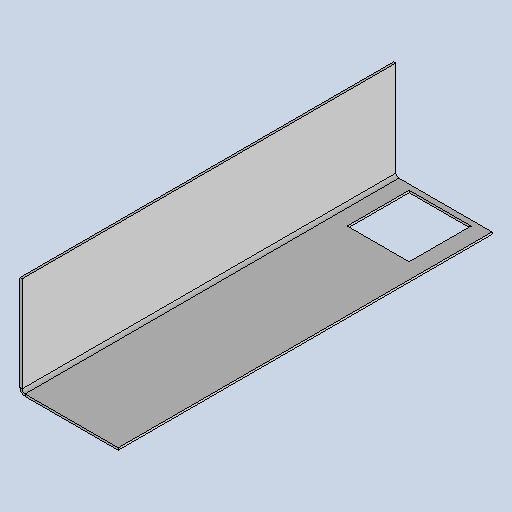
# Autodesk Inventor part: PNS 752 FDS 1200 FLANGE 2_1600
Saved by Autodesk Inventor 2025 (Build 290162010, 162A)
## iProperties
Created: 2025-06-24
Part Number: PNS 752 FDS 1200 FLANGE 2_1600
Material: Stainless Steel
Description: DIE16(5)|\ 90°|corrY -___°|X_____|bom___
Document SubType Name: Sheet Metal
Designer: admin
Mass: 967.563 g
Surface Area: 1235.39 cm^2
Volume: 120.945 cm^3
Density: 8 g/cm^3
Flat Pattern Width: 18.2202 cm
Flat Pattern Length: 35 cm
Flat Pattern Area: 637.707 cm^2
Sheet Metal Rule: AISI304 2mm Die16
Sheet Metal Width: 182.202 mm
Sheet Metal Length: 350.000 mm
Sheet Metal Area: 63770.697 mm^2
Appearance: Default
Author: user
Autodesk Inventor part; units mm, degrees
ref_plane "YZ Plane" through (0, 0, 0) normal (1, 0, 0) x (0, 1, 0)
ref_plane "XZ Plane" through (0, 0, 0) normal (0, 1, 0) x (-1, 0, 0)
ref_plane "XY Plane" through (0, 0, 0) normal (0, 0, 1) x (1, 0, 0)
sketch "Sketch1" plane through (0, 0, 0) normal (0, 0, 1) x (1, 0, 0)
  line L0 (-46, -175) -> (46, -175)
  line L1 (46, -175) -> (46, 175)
  line L2 (46, 175) -> (-46, 175)
  line L3 (-46, 175) -> (-46, -175)
  line L4 (-46, -175) -> (46, 175) construction
  line L5 (46, -175) -> (-46, 175) construction
  point P0 (0, 0)
  dimension "d154" = 92
  dimension "d155" = 350
  measures "d154" distance of L1.end L2.end
  measures "d155" distance of L0.end L1.end
extrude "Plate5" add sketch "Sketch1" along normal blind 2
sketch "Sketch7" plane through (-44, -175, 0) normal (-1, 0, 0) x (0, -1, 0)
  line L0 (-350, 0) -> (0, 0)
  line L1 (0, 0) -> (0, 94)
  line L2 (0, 94) -> (-350, 94)
  line L3 (-350, 94) -> (-350, 0)
  constraints: 6 end point, 1 horizontal, 1 perpendicular, 1 vertical
edge flange "Flange3" height 94 angle 90 thickness 2 bend radius 2.75 thickness toward (-1, 0, 0) relief round relief width 2 relief depth 1 edges at (-46, 0, 2) wall of the first edge with corners at (-44, 175, 0) (-44, -175, 0) (-44, -175, 94) (-44, 175, 94)
bend "Bend3"
corner "Corner3"
sketch "Sketch8" plane through (0, 0, 2) normal (0, 0, 1) x (1, 0, 0)
  line L0 (46, 175) -> (46, -175) projected
  line L1 (-41.25, 175) -> (46, 175) projected
  line L2 (31.375, 170) -> (-26.625, 170)
  line L3 (-26.625, 170) -> (-26.625, 112)
  line L4 (-26.625, 112) -> (31.375, 112)
  line L5 (31.375, 112) -> (31.375, 170)
  line L6 (31.375, 170) -> (-26.625, 112) construction
  line L7 (-26.625, 170) -> (31.375, 112) construction
  point P0 (0, 0)
  point P1 (2.375, 141)
  point P2 (2.375, 175)
  dimension "d167" = 58
  dimension "d168" = 58
  dimension "d169" = 5
  constraints: 12 end point, 3 midpoint, 2 parallel, 1 horizontal, 1 perpendicular, 1 vertical alignment
  measures "d167" distance of L4.end L3.end
  measures "d168" distance of L3.end L2.end
  measures "d169" distance between parallel lines of L1 L2
extrude "Cut1" cut sketch "Sketch8" against normal blind 2
body "Solid3"
